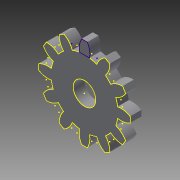
# Autodesk Inventor part: Sun
Saved by Autodesk Inventor 2013 (Build 170138000, 138)
## iProperties
Created: 2014-02-12
Part Number: Sun
Material: Generic
Document SubType Name: Modeling
Designer: robotics
Density: 1 g/cm^3
Author: robotics
Autodesk Inventor part; units mm, degrees
ref_plane "YZ Plane" through (0, 0, 0) normal (1, 0, 0) x (0, 1, 0)
ref_plane "XZ Plane" through (0, 0, 0) normal (0, 1, 0) x (-1, 0, 0)
ref_plane "XY Plane" through (0, 0, 0) normal (0, 0, 1) x (1, 0, 0)
sketch "Sketch1" plane through (0, 0, 0) normal (0, 0, 1) x (1, 0, 0)
  line L0 (0, 0) -> (0, 20.872) construction
  line L1 (0, 0) -> (7.1878, 0) construction
  line L2 (0, 6.45) -> (0.3969, 6.45)
  line L3 (0.3969, 6.45) -> (0.71, 4.674) construction
  line L4 (0.5535, 5.562) -> (2.6468, 5.9311) construction
  arc A0 (0.71, 4.674) -> (0.3969, 6.45) centre (-1.785, 5.1496) ccw
  line L5 (0, 6.45) -> (-0.3969, 6.45)
  arc A1 (-0.3969, 6.45) -> (-0.71, 4.674) centre (1.785, 5.1496) ccw
  line L6 (-0.3969, 6.45) -> (0.3969, 6.45)
  line L7 (-0.3969, 6.45) -> (0.3969, 6.45)
  line L8 (-3.225, 5.5858) -> (-2.8813, 5.7843)
  arc A2 (-1.7221, 4.4028) -> (-2.8813, 5.7843) centre (-4.1207, 3.5672) ccw
  arc A3 (-3.5687, 5.3874) -> (-2.9519, 3.6928) centre (-1.0289, 5.3522) ccw
  line L9 (-3.225, 5.5858) -> (-3.5687, 5.3874)
  line L10 (-5.5858, 3.225) -> (-5.3874, 3.5687)
  arc A4 (-3.6928, 2.9519) -> (-5.3874, 3.5687) centre (-5.3522, 1.0289) ccw
  arc A5 (-5.7843, 2.8813) -> (-4.4028, 1.7221) centre (-3.5672, 4.1207) ccw
  line L11 (-5.5858, 3.225) -> (-5.7843, 2.8813)
  line L12 (-6.45, 0) -> (-6.45, 0.3969)
  arc A6 (-4.674, 0.71) -> (-6.45, 0.3969) centre (-5.1496, -1.785) ccw
  arc A7 (-6.45, -0.3969) -> (-4.674, -0.71) centre (-5.1496, 1.785) ccw
  line L13 (-6.45, 0) -> (-6.45, -0.3969)
  line L14 (-5.5858, -3.225) -> (-5.7843, -2.8813)
  arc A8 (-4.4028, -1.7221) -> (-5.7843, -2.8813) centre (-3.5672, -4.1207) ccw
  arc A9 (-5.3874, -3.5687) -> (-3.6928, -2.9519) centre (-5.3522, -1.0289) ccw
  line L15 (-5.5858, -3.225) -> (-5.3874, -3.5687)
  line L16 (-3.225, -5.5858) -> (-3.5687, -5.3874)
  arc A10 (-2.9519, -3.6928) -> (-3.5687, -5.3874) centre (-1.0289, -5.3522) ccw
  arc A11 (-2.8813, -5.7843) -> (-1.7221, -4.4028) centre (-4.1207, -3.5672) ccw
  line L17 (-3.225, -5.5858) -> (-2.8813, -5.7843)
  line L18 (0, -6.45) -> (-0.3969, -6.45)
  arc A12 (-0.71, -4.674) -> (-0.3969, -6.45) centre (1.785, -5.1496) ccw
  arc A13 (0.3969, -6.45) -> (0.71, -4.674) centre (-1.785, -5.1496) ccw
  line L19 (0, -6.45) -> (0.3969, -6.45)
  line L20 (3.225, -5.5858) -> (2.8813, -5.7843)
  arc A14 (1.7221, -4.4028) -> (2.8813, -5.7843) centre (4.1207, -3.5672) ccw
  arc A15 (3.5687, -5.3874) -> (2.9519, -3.6928) centre (1.0289, -5.3522) ccw
  line L21 (3.225, -5.5858) -> (3.5687, -5.3874)
  line L22 (5.5858, -3.225) -> (5.3874, -3.5687)
  arc A16 (3.6928, -2.9519) -> (5.3874, -3.5687) centre (5.3522, -1.0289) ccw
  arc A17 (5.7843, -2.8813) -> (4.4028, -1.7221) centre (3.5672, -4.1207) ccw
  line L23 (5.5858, -3.225) -> (5.7843, -2.8813)
  line L24 (6.45, 0) -> (6.45, -0.3969)
  arc A18 (4.674, -0.71) -> (6.45, -0.3969) centre (5.1496, 1.785) ccw
  arc A19 (6.45, 0.3969) -> (4.674, 0.71) centre (5.1496, -1.785) ccw
  line L25 (6.45, 0) -> (6.45, 0.3969)
  line L26 (5.5858, 3.225) -> (5.7843, 2.8813)
  arc A20 (4.4028, 1.7221) -> (5.7843, 2.8813) centre (3.5672, 4.1207) ccw
  arc A21 (5.3874, 3.5687) -> (3.6928, 2.9519) centre (5.3522, 1.0289) ccw
  line L27 (5.5858, 3.225) -> (5.3874, 3.5687)
  line L28 (3.225, 5.5858) -> (3.5687, 5.3874)
  arc A22 (2.9519, 3.6928) -> (3.5687, 5.3874) centre (1.0289, 5.3522) ccw
  arc A23 (2.8813, 5.7843) -> (1.7221, 4.4028) centre (4.1207, 3.5672) ccw
  line L29 (3.225, 5.5858) -> (2.8813, 5.7843)
  line L30 (-1.7221, 4.4028) -> (-0.71, 4.674) construction
  arc A24 (1.7221, 4.4028) -> (0.71, 4.674) centre (0, 0) ccw
  arc A25 (3.6928, 2.9519) -> (2.9519, 3.6928) centre (0, 0) ccw
  arc A26 (4.674, 0.71) -> (4.4028, 1.7221) centre (0, 0) ccw
  arc A27 (4.4028, -1.7221) -> (4.674, -0.71) centre (0, 0) ccw
  arc A28 (2.9519, -3.6928) -> (3.6928, -2.9519) centre (0, 0) ccw
  arc A29 (0.71, -4.674) -> (1.7221, -4.4028) centre (0, 0) ccw
  arc A30 (-1.7221, -4.4028) -> (-0.71, -4.674) centre (0, 0) ccw
  arc A31 (-3.6928, -2.9519) -> (-2.9519, -3.6928) centre (0, 0) ccw
  arc A32 (-4.674, -0.71) -> (-4.4028, -1.7221) centre (0, 0) ccw
  arc A33 (-4.4028, 1.7221) -> (-4.674, 0.71) centre (0, 0) ccw
  arc A34 (-0.71, 4.674) -> (-1.7221, 4.4028) centre (0, 0) ccw
  arc A35 (-2.9519, 3.6928) -> (-3.6928, 2.9519) centre (0, 0) ccw
  dimension "d0" = 0.7937
  dimension "d4" = 360
  dimension "d6" = 80
  dimension "d7" = 1.8034
  dimension "d8" = 2.54
  dimension "d11" = 1.0477
  constraints: 72 point on circle, 62 end point, 36 centre point, 3 symmetric about line, 2 collinear, 2 perpendicular, 1 coincident, 1 midpoint, 1 parallel, 1 point on line, 1 vertical, 134 other
  measures "d0" distance of L5.end L2.end
  measures "d6" angle of L1 L3
  measures "d7" distance of L2.end L3.end
  measures "d8" radius of A0
  measures "d11" distance of L30.start L30.end
extrude "Extrusion1" add sketch "Sketch1" along normal blind 1.5875
sketch "Sketch2" plane through (0, 0, 1.5875) normal (0, 0, 1) x (1, 0, 0)
  arc A0 (1.7221, 4.4028) -> (0.71, 4.674) centre (0, 0) ccw projected
  circle A1 centre (0, 0) radius 1.5875
  dimension "d12" = 3.175
  constraints: 1 centre point, 1 coincident
  measures "d12" diameter of A1
extrude "Extrusion2" cut sketch "Sketch2" against normal blind 1.5875
sketch "Sketch3" plane through (0, 0, 1.5875) normal (0, 0, 1) x (1, 0, 0)
  circle A0 centre (0, 0) radius 1.5875 projected
  arc A1 (-0.3969, 6.45) -> (-0.71, 4.674) centre (1.785, 5.1496) ccw projected
  arc A2 (-0.71, 4.674) -> (-1.7221, 4.4028) centre (0, 0) ccw projected
  arc A3 (-1.7221, 4.4028) -> (-2.8813, 5.7843) centre (-4.1207, 3.5672) ccw projected
  line L0 (-2.8813, 5.7843) -> (-3.5687, 5.3874) projected
  arc A4 (-3.5687, 5.3874) -> (-2.9519, 3.6928) centre (-1.0289, 5.3522) ccw projected
  arc A5 (-2.9519, 3.6928) -> (-3.6928, 2.9519) centre (0, 0) ccw projected
  arc A6 (-3.6928, 2.9519) -> (-5.3874, 3.5687) centre (-5.3522, 1.0289) ccw projected
  line L1 (-5.3874, 3.5687) -> (-5.7843, 2.8813) projected
  arc A7 (-5.7843, 2.8813) -> (-4.4028, 1.7221) centre (-3.5672, 4.1207) ccw projected
  arc A8 (-4.4028, 1.7221) -> (-4.674, 0.71) centre (0, 0) ccw projected
  arc A9 (-4.674, 0.71) -> (-6.45, 0.3969) centre (-5.1496, -1.785) ccw projected
  line L2 (-6.45, 0.3969) -> (-6.45, -0.3969) projected
  arc A10 (-6.45, -0.3969) -> (-4.674, -0.71) centre (-5.1496, 1.785) ccw projected
  arc A11 (-4.674, -0.71) -> (-4.4028, -1.7221) centre (0, 0) ccw projected
  arc A12 (-4.4028, -1.7221) -> (-5.7843, -2.8813) centre (-3.5672, -4.1207) ccw projected
  line L3 (-5.7843, -2.8813) -> (-5.3874, -3.5687) projected
  arc A13 (-5.3874, -3.5687) -> (-3.6928, -2.9519) centre (-5.3522, -1.0289) ccw projected
  arc A14 (-3.6928, -2.9519) -> (-2.9519, -3.6928) centre (0, 0) ccw projected
  arc A15 (-2.9519, -3.6928) -> (-3.5687, -5.3874) centre (-1.0289, -5.3522) ccw projected
  line L4 (-3.5687, -5.3874) -> (-2.8813, -5.7843) projected
  arc A16 (-2.8813, -5.7843) -> (-1.7221, -4.4028) centre (-4.1207, -3.5672) ccw projected
  arc A17 (-1.7221, -4.4028) -> (-0.71, -4.674) centre (0, 0) ccw projected
  arc A18 (-0.71, -4.674) -> (-0.3969, -6.45) centre (1.785, -5.1496) ccw projected
  line L5 (-0.3969, -6.45) -> (0.3969, -6.45) projected
  arc A19 (0.3969, -6.45) -> (0.71, -4.674) centre (-1.785, -5.1496) ccw projected
  arc A20 (0.71, -4.674) -> (1.7221, -4.4028) centre (0, 0) ccw projected
  arc A21 (1.7221, -4.4028) -> (2.8813, -5.7843) centre (4.1207, -3.5672) ccw projected
  line L6 (2.8813, -5.7843) -> (3.5687, -5.3874) projected
  arc A22 (3.5687, -5.3874) -> (2.9519, -3.6928) centre (1.0289, -5.3522) ccw projected
  arc A23 (2.9519, -3.6928) -> (3.6928, -2.9519) centre (0, 0) ccw projected
  arc A24 (3.6928, -2.9519) -> (5.3874, -3.5687) centre (5.3522, -1.0289) ccw projected
  line L7 (5.3874, -3.5687) -> (5.7843, -2.8813) projected
  arc A25 (5.7843, -2.8813) -> (4.4028, -1.7221) centre (3.5672, -4.1207) ccw projected
  arc A26 (4.4028, -1.7221) -> (4.674, -0.71) centre (0, 0) ccw projected
  arc A27 (4.674, -0.71) -> (6.45, -0.3969) centre (5.1496, 1.785) ccw projected
  line L8 (6.45, -0.3969) -> (6.45, 0.3969) projected
  arc A28 (6.45, 0.3969) -> (4.674, 0.71) centre (5.1496, -1.785) ccw projected
  arc A29 (4.674, 0.71) -> (4.4028, 1.7221) centre (0, 0) ccw projected
  arc A30 (4.4028, 1.7221) -> (5.7843, 2.8813) centre (3.5672, 4.1207) ccw projected
  line L9 (5.7843, 2.8813) -> (5.3874, 3.5687) projected
  arc A31 (5.3874, 3.5687) -> (3.6928, 2.9519) centre (5.3522, 1.0289) ccw projected
  arc A32 (3.6928, 2.9519) -> (2.9519, 3.6928) centre (0, 0) ccw projected
  arc A33 (2.9519, 3.6928) -> (3.5687, 5.3874) centre (1.0289, 5.3522) ccw projected
  line L10 (3.5687, 5.3874) -> (2.8813, 5.7843) projected
  arc A34 (2.8813, 5.7843) -> (1.7221, 4.4028) centre (4.1207, 3.5672) ccw projected
  arc A35 (1.7221, 4.4028) -> (0.71, 4.674) centre (0, 0) ccw projected
  arc A36 (0.71, 4.674) -> (0.3969, 6.45) centre (-1.785, 5.1496) ccw projected
  line L11 (0.3969, 6.45) -> (-0.3969, 6.45) projected
  line L12 (-0.71, 4.674) -> (0.71, 4.674)
  arc A37 (0.71, 4.674) -> (0.3969, 6.45) centre (-1.785, 5.1496) ccw
  line L13 (0.3969, 6.45) -> (-0.3969, 6.45)
  arc A38 (-0.3969, 6.45) -> (-0.71, 4.674) centre (1.785, 5.1496) ccw
  constraints: 4 end point, 4 point on circle, 2 centre point, 2 concentric, 1 collinear, 1 parallel
body "Solid1"
